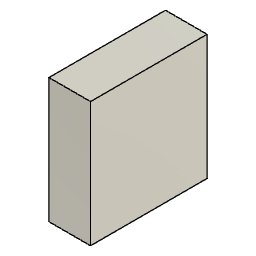
unsorted_smarties_holder_support (Autodesk Fusion 360 design; units mm, degrees)
Autodesk Fusion 360 part; units mm, degrees
sketch "Unsorted Smarties Holder Support" plane through (0, 0, 0) normal (0, 0, 1) x (1, 0, 0)
  line L0 (0, 0) -> (-10, 0)
  line L1 (-10, 0) -> (-10, 28)
  line L2 (-10, 28) -> (0, 28)
  line L3 (0, 28) -> (0, 0)
  dimension "d1" = 10
  dimension "d2" = 28
  constraint horizontal L0
  constraint vertical L1
  constraint horizontal L2
  constraint vertical L3
  constraint coincident L0.start L3.end
  measures "d1" distance of L0.start L0.end
  measures "d2" distance of L0.start L2.end
extrude "Extrude1" add sketch "Unsorted Smarties Holder Support" along normal blind 30
named bodies: "Unsorted Smarties Holder Support"
